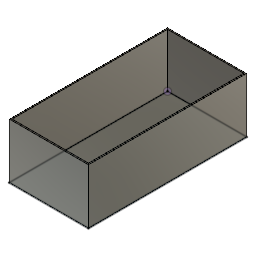
CircuitCase_v3 (Autodesk Fusion 360 design; units mm, degrees)
Autodesk Fusion 360 part; units mm, degrees
sketch "Sketch3" plane through (0, 0, 0) normal (0, 0, 1) x (1, 0, 0)
  line L0 (0, 0) -> (57.5, 0)
  line L1 (57.5, 0) -> (57.5, -115)
  line L2 (57.5, -115) -> (0, -115)
  line L3 (0, -115) -> (0, 0)
  dimension "d4" = 57.5
  dimension "d5" = 115
  constraint horizontal L0
  constraint vertical L1
  constraint horizontal L2
  constraint vertical L3
  constraint coincident L0.start L3.end
  measures "d4" distance of L0.start L0.end
  measures "d5" distance of L0.start L2.end
sketch "Sketch4" plane through (0, 0, 0) normal (0, 0, 1) x (1, 0, 0)
extrude "Extrude1" add sketch "Sketch3" along normal blind 40
sketch "Sketch5" plane through (0, -115, 0) normal (0, -1, 0) x (1, 0, 0)
  line L0 (0, 0) -> (57.5, 0)
  line L1 (57.5, 0) -> (57.5, 40)
  line L2 (57.5, 40) -> (0, 40)
  line L3 (0, 40) -> (0, 0)
shell "Shell1" thickness 1 removed faces 1 at (19.1667, -38.3333, 40)
sketch "Sketch7" plane through (0, 0, 1) normal (0, 0, 1) x (-1, 0, 0)
  line L0 (-1, 114) -> (-56.5, 114)
  line L1 (-56.5, 114) -> (-56.5, 1)
  line L2 (-56.5, 1) -> (-1, 1)
  line L3 (-1, 1) -> (-1, 114)
  line L4 (-14.7329, 75.3584) -> (-40.1329, 75.3584)
  line L5 (-40.1329, 75.3584) -> (-40.1329, 100.7584)
  line L6 (-40.1329, 100.7584) -> (-14.7329, 100.7584)
  line L7 (-14.7329, 100.7584) -> (-14.7329, 75.3584)
  dimension "d9" = 25.4
  dimension "d10" = 25.4
  constraint horizontal L4
  constraint vertical L5
  constraint horizontal L6
  constraint vertical L7
  measures "d9" distance of L4.start L4.end
  measures "d10" distance of L4.start L6.end
extrude "Extrude2" cut sketch "Sketch7" against normal blind 10 contours L4 L5 L6 L7
